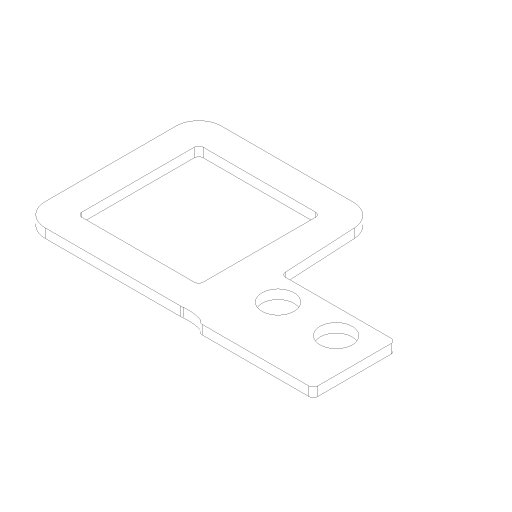
# Autodesk Inventor part: PCB_arm
Saved by Autodesk Inventor 2023 (Build 270158000, 158)
## iProperties
Created: 2024-03-15
Part Number: PCB_arm
Material: Generic
Document SubType Name: Modeling
Designer: ferrerx
Density: 1 g/cm^3
Appearance: Default
Author: ferrerx
Autodesk Inventor part; units mm, degrees
ref_plane "YZ Plane" through (0, 0, 0) normal (1, 0, 0) x (0, 1, 0)
ref_plane "XZ Plane" through (0, 0, 0) normal (0, 1, 0) x (-1, 0, 0)
ref_plane "XY Plane" through (0, 0, 0) normal (0, 0, 1) x (1, 0, 0)
sketch "Sketch1" plane through (0, 0, 0) normal (0, 1, 0) x (-1, 0, 0)
  line L0 (5, -3.567) -> (5, 0.033)
  line L1 (5, 0.033) -> (0, 0.033)
  line L2 (5.2265, -7.8894) -> (5, -3.567)
  line L3 (5.2265, -0.5894) -> (5, 0.033)
  line L4 (0, -3.567) -> (0, 0.033)
  line L5 (5, -3.567) -> (0, -3.567)
  line L6 (5.2265, -0.1894) -> (12.9265, -0.1894)
  line L7 (12.9265, -0.1894) -> (12.9265, -7.8894)
  line L8 (12.9265, -7.8894) -> (5.2265, -7.8894)
  line L9 (5.2265, -7.8894) -> (5.2265, -0.1894)
  line L10 (5.2265, -0.5894) -> (5.2265, -7.8894) construction
  line L11 (5.2265, -4.2394) -> (11.8919, -4.2394) construction
  line L12 (11.7265, -6.6894) -> (6.4265, -6.6894)
  line L13 (6.4265, -6.6894) -> (6.4265, -1.3894)
  line L14 (6.4265, -1.3894) -> (11.7265, -1.3894)
  line L15 (11.7265, -1.3894) -> (11.7265, -6.6894)
  point P0 (6.1218, -0.1118)
  point P1 (5.2265, -0.5894)
  point P2 (5.4261, -0.5894)
  dimension "d9" = 3.6
  dimension "d10" = 160
  dimension "d12" = 93
  dimension "d18" = 3.65
  dimension "d20" = 1.2
  dimension "d22" = 1.2
  dimension "d28" = 5
  dimension "d39" = 5.3
  dimension "d40" = 5.3
  dimension "d41" = 1.2
  dimension "d42" = 1.2
  constraints: 33 end point, 5 parallel, 4 horizontal, 3 perpendicular, 2 vertical, 1 midpoint, 1 vertical alignment, 2 other
  measures "d9" distance of L4.start L1.end
  measures "d10" angle of L0 L3
  measures "d12" angle of L5 L2
  measures "d18" distance between parallel lines of L8 L11
  measures "d20" distance between parallel lines of L7 L15
  measures "d22" distance between parallel lines of L9 L13
  measures "d28" distance between parallel lines of L4 L0
  measures "d39" distance of L14.end L12.start
  measures "d40" distance of L13.end L14.end
  measures "d41" distance between parallel lines of L8 L12
  measures "d42" distance between parallel lines of L6 L14
extrude "Extrusion1" add sketch "Sketch1" along normal blind 0.4
fillet "Fillet3" radius 1 4 edges at (-12.9265, 0.2, -0.1894) (-5.2265, 0.2, -0.1894) (-5.2265, 0.2, -7.8894) (-12.9265, 0.2, -7.8894)
fillet "Fillet4" radius 0.2 4 edges at (-6.4265, 0.2, -6.6894) (-11.7265, 0.2, -6.6894) (-11.7265, 0.2, -1.3894) (-6.4265, 0.2, -1.3894)
fillet "Fillet6" radius 0.2 4 edges at (-5, 0.2, 0.033) (0, 0.2, 0.033) (0, 0.2, -3.567) (-5, 0.2, -3.567)
sketch "Sketch2" plane through (0, 0.4, 0) normal (0, 1, 0) x (1, 0, 0)
  line L0 (0, 0.167) -> (0, 3.367) projected
  circle A0 centre (-4.04, 2.467) radius 0.7
  circle A1 centre (-1.5, 2.467) radius 0.7
  line L1 (-4.04, 2.467) -> (-1.5, 2.467) construction
  line L2 (-4.86, -0.033) -> (-0.2, -0.033) projected
  line L3 (-0.2, 3.567) -> (-4.8102, 3.567) projected
  point P0 (0, 0)
  dimension "d29" = 1.4
  dimension "d31" = 2.54
  dimension "d32" = 1.5
  dimension "d38" = 1.1
  constraints: 2 centre point, 2 end point, 1 equal radius, 1 horizontal
  measures "d29" diameter of A0
  measures "d31" distance of L1.end L1.start
  measures "d32" distance from line of L0 L1.end
  measures "d38" distance between parallel lines of L3 L1
extrude "Extrusion2" cut sketch "Sketch2" against normal blind 0.4
fillet "Fillet8" [suppressed]
fillet "Fillet9" radius 2 1 edges at (-5.2265, 0.2, -0.5894)
equation "\"d18\" = 0.5 * d15"
equation "\"d15\" = 7.3"
body "Solid1"
